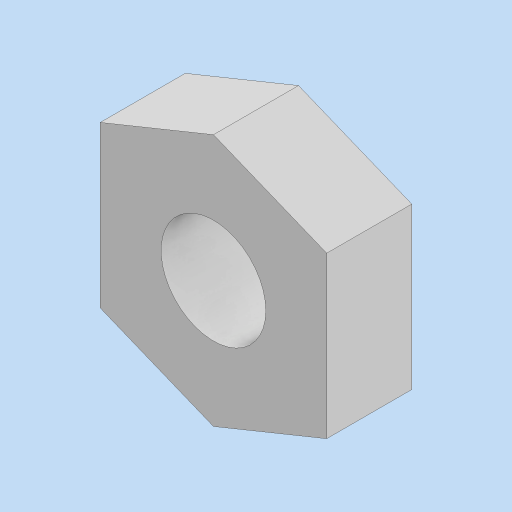
# Autodesk Inventor part: tuerca2mockup
Saved by Autodesk Inventor 2024 (Build 280153000, 153)
## iProperties
Created: 2024-09-12
Part Number: tuerca2mockup
Material: Generic
Document SubType Name: Modeling
Designer: MxMon
Density: 1 g/cm^3
Appearance: Default
Author: MxMon
Autodesk Inventor part; units mm, degrees
ref_plane "YZ Plane" through (0, 0, 0) normal (1, 0, 0) x (0, 1, 0)
ref_plane "XZ Plane" through (0, 0, 0) normal (0, 1, 0) x (-1, 0, 0)
ref_plane "XY Plane" through (0, 0, 0) normal (0, 0, 1) x (1, 0, 0)
sketch "Sketch1" plane through (0, 0, 0) normal (0, 0, 1) x (1, 0, 0)
  circle A0 centre (0, 0) radius 2
  line L0 (0, 4.825) -> (-4.325, 3.0677)
  line L1 (-4.325, 3.0677) -> (-4.325, -3.0677)
  line L2 (-4.325, -3.0677) -> (0, -4.825)
  line L3 (0, -4.825) -> (4.325, -3.0677)
  line L4 (4.325, -3.0677) -> (4.325, 3.0677)
  line L5 (4.325, 3.0677) -> (0, 4.825)
  line L6 (-4.325, 0) -> (4.325, 0)
  arc A1 (-2, 0) -> (2, 0) centre (0, 0) ccw
  arc A2 (2, 0) -> (-2, 0) centre (0, 0) ccw
  point P0 (0, 0)
  point P1 (-1.781, -6.0193)
  point P2 (0, 0)
  dimension "d0" = 9
  dimension "d1" = 8.65
  dimension "d2" = 9.65
  dimension "d3" = 9
  dimension "d4" = 4
  constraints: 14 end point, 6 point on circle, 3 centre point, 3 equal length, 3 midpoint, 2 concentric, 2 parallel, 2 point on line, 1 coincident, 1 horizontal alignment, 1 vertical, 1 vertical alignment
  measures "d0" distance of L0.start L1.end
  measures "d1" distance between parallel lines of L4 L1
  measures "d2" distance of L2.end L0.start
  measures "d3" distance of L0.start L3.end
  measures "d4" diameter of A0
extrude "Extrusion1" add sketch "Sketch1" along normal blind 3.25 contours L6 L4 L3 L2 L1 A0 | A0 L6 L1 L0 L5 L4
body "Solid1"
